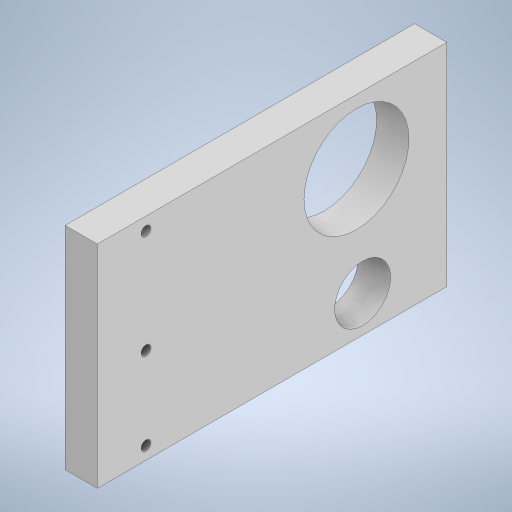
# Autodesk Inventor part: Frame Sides
Saved by Autodesk Inventor 2023 (Build 270158000, 158)
## iProperties
Created: 2022-12-23
Part Number: Frame Sides
Material: Generic
Document SubType Name: Modeling
Designer: tgr41
Density: 1 g/cm^3
Appearance: Default
Author: tgr41
Autodesk Inventor part; units mm, degrees
ref_plane "YZ Plane" through (0, 0, 0) normal (1, 0, 0) x (0, 1, 0)
ref_plane "XZ Plane" through (0, 0, 0) normal (0, 1, 0) x (-1, 0, 0)
ref_plane "XY Plane" through (0, 0, 0) normal (0, 0, 1) x (1, 0, 0)
sketch "Sketch1" plane through (0, 0, 0) normal (1, 0, 0) x (0, 1, 0)
  circle A0 centre (5.08, -11.43) radius 1.905
  circle A1 centre (78.105, -11.43) radius 1.905
  circle A2 centre (37.465, -11.43) radius 1.905
  line L0 (83.185, -17.78) -> (83.185, 7.62)
  line L1 (83.185, 7.62) -> (0, 7.62)
  line L2 (0, 7.62) -> (0, -129.794)
  line L3 (83.185, 7.62) -> (83.185, 4.445)
  line L4 (83.185, 7.62) -> (83.185, -129.794)
  line L5 (83.185, -129.794) -> (0, -129.794)
  circle A3 centre (57.785, -94.234) radius 20.6375
  circle A4 centre (14.2875, -96.6479) radius 10.9982
  point P0 (0, 0)
  dimension "d16" = 3.81
  dimension "d51" = 3.81
  dimension "d52" = 3.81
  dimension "d53" = 137.414
  dimension "d54" = 41.275
  dimension "d55" = 21.9964
  dimension "d56" = 19.05
  dimension "d57" = 19.05
  dimension "d58" = 19.05
  dimension "d59" = 5.08
  dimension "d60" = 37.465
  dimension "d61" = 78.105
  dimension "d62" = 101.854
  dimension "d63" = 104.2679
  dimension "d64" = 25.4
  dimension "d65" = 14.2875
  dimension "d66" = 83.185
  constraints: 12 end point, 5 centre point, 1 horizontal, 1 perpendicular, 1 point on line, 1 vertical
  measures "d16" diameter of A0
  measures "d51" diameter of A2
  measures "d52" diameter of A1
  measures "d53" distance of L0.end L4.end
  measures "d54" diameter of A3
  measures "d55" diameter of A4
  measures "d56" distance from line of L1 A1.centre
  measures "d57" distance from line of L1 A2.centre
  measures "d58" distance from line of L1 A0.centre
  measures "d59" distance from line of L2 A0.centre
  measures "d60" distance from line of L2 A2.centre
  measures "d61" distance from line of L2 A1.centre
  measures "d62" distance from line of L1 A3.centre
  measures "d63" distance from line of L1 A4.centre
  measures "d64" distance from line of L4 A3.centre
  measures "d65" distance from line of L2 A4.centre
  measures "d66" distance between parallel lines of L2 L4
extrude "Extrusion6" add sketch "Sketch1" along normal blind 12.7
body "Solid3"
